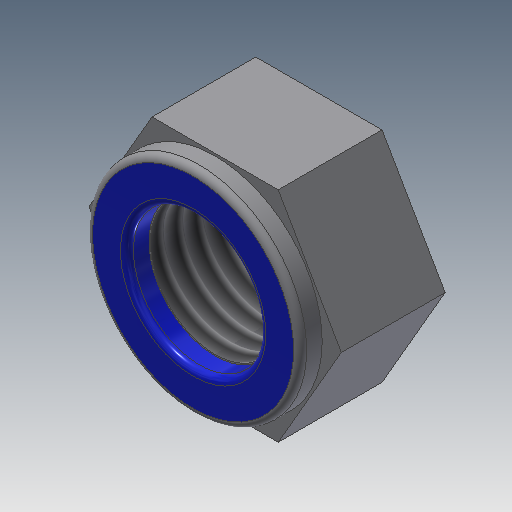
# Autodesk Inventor part: M10 Nut (o'ring)
Saved by Autodesk Inventor 2018 (Build 220112000, 112)
## iProperties
Shininess: 64.0
Length Units: 11269
Angle Units: 11279
Time Units: 11290
Mass Units: 11283
Length Display Precision: 3
Angle Display Precision: 2
Compacted: True
Part Number: M10 Nut (o'ring)
Document SubType Name: Modeling
Created: 2003-03-27
Designer: ASUS1
Material: Generic
Density: 1 g/cm^3
Appearance: Default
Density: 0.0
Volumn: 0.0
Area: 0.0
PropertySet Name: Model Information
Control State: 0
Master: False
Checked Out: False
Author: ASUS1
Autodesk Inventor part; units mm, degrees
ref_plane "YZ Plane" through (0, 0, 0) normal (1, 0, 0) x (0, 1, 0)
ref_plane "XZ Plane" through (0, 0, 0) normal (0, 1, 0) x (-1, 0, 0)
sketch "Sketch1" plane through (0, 0, 0) normal (0, 0, 1) x (1, 0, 0)
  circle A0 centre (34.0098, 33.0258) radius 5
  circle A1 centre (34.0098, 33.0258) radius 8.425
  line L0 (38.874, 41.4508) -> (43.7382, 33.0258)
  line L1 (43.7382, 33.0258) -> (38.874, 24.6008)
  line L2 (38.874, 24.6008) -> (29.1457, 24.6008)
  line L3 (29.1457, 24.6008) -> (24.2815, 33.0258)
  line L4 (24.2815, 33.0258) -> (29.1457, 41.4508)
  line L5 (29.1457, 41.4508) -> (38.874, 41.4508)
  point P0 (34.0098, 41.4508)
  dimension "d1" = 16.85
  dimension "d0" = 10
  constraints: 12 end point, 2 coincident, 1 centre point, 1 midpoint, 1 vertical alignment, 14 other
  measures "d0" diameter of A0
extrude "Extrusion1" add sketch "Sketch1" along normal blind 8
ref_plane "Work Plane1" through (34.0098, 33.0258, 0) normal (0.866, -0.5, 0) x (0, 0, 1)
thread "Thread1" size "M10x1.5" class "6H" standard "ANSI Metric M Profile" full length
sketch "Sketch4" plane through (0, 0, 8) normal (0, 0, 1) x (1, 0, 0)
  circle A0 centre (34.0098, 33.0258) radius 5 projected
  circle A1 centre (34.0098, 33.0258) radius 8.25
  circle A2 centre (34.0098, 33.0258) radius 5.1
  dimension "d11" = 16.5
  dimension "d12" = 10.2
  constraints: 2 centre point, 2 concentric
  measures "d11" diameter of A1
  measures "d12" diameter of A2
extrude "Extrusion2" add sketch "Sketch4" along normal blind 1.7 contours A1
fillet "Fillet1" radius 0.5 2 edges at (28.9098, 33.0258, 9.7) (25.7598, 33.0258, 9.7)
body "Solid1"
